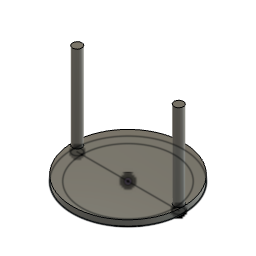
ball_release_node_01 (Autodesk Fusion 360 design; units mm, degrees)
Autodesk Fusion 360 part; units mm, degrees
sketch "Sketch1" plane through (0, 0, 0) normal (0, 1, 0) x (1, 0, 0)
  circle A0 centre (0, 0) radius 7.9375
  line L0 (0, 0) -> (7.9375, 0)
  line L1 (0, 0) -> (-7.9375, 0)
  line L2 (-7.9375, 0) -> (-8.7313, 0)
  circle A1 centre (-8.7313, 0) radius 0.7937
  line L3 (7.9375, 0) -> (8.7313, 0)
  circle A2 centre (8.7313, 0) radius 0.7937
  circle A3 centre (0, 0) radius 9.525
  dimension "d1" = 15.875
  dimension "d4" = 0.7937
  dimension "d5" = 1.5875
  dimension "d6" = 0.7937
  dimension "d7" = 1.5875
  constraint coincident A0.centre L0.start
  constraint coincident A0 L0.end
  constraint horizontal L0
  constraint coincident A0 L1.end
  constraint parallel L0 L1
  constraint parallel L1 L2
  constraint coincident L2.end A1.centre
  constraint parallel L0 L3
  constraint coincident L3.end A2.centre
  constraint concentric A0 A3
  constraint tangent A2 A3
  measures "d1" diameter of A0
  measures "d4" distance of L1.end L2.end
  measures "d5" diameter of A1
  measures "d6" distance of L0.end L3.end
  measures "d7" diameter of A2
extrude "Extrude1" add sketch "Sketch1" along normal blind 1 contours A0 L0 L1 | A0 A1 A2 A3 | A0 L0 L1 | A0 A1 A2 A3
extrude "Extrude2" add sketch "Sketch1" along normal blind 15.875 contours A2 | A1
equation "d4 = ( 1.5875 / 2 ) * 1 mm"
equation "d6 = ( 1.5875 / 2 ) * 1 mm"
